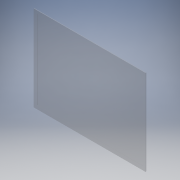
# Autodesk Inventor part: resistive_panel_12.1
Saved by Autodesk Inventor 2017 (Build 210142000, 142)
## iProperties
Created: 2017-04-25
Part Number: resistive_panel_12.1
Material: Szkło
Document SubType Name: Modeling
Designer: Speed King
Density: 2.18 g/cm^3
Appearance: Poliwęglan — przezroczysty
Mass: 270.887 g
Surface Area: 1618.77 cm^2
Volume: 124.26 cm^3
Author: Speed King
Autodesk Inventor part; units mm, degrees
ref_plane "YZ Plane" through (0, 0, 0) normal (1, 0, 0) x (0, 1, 0)
ref_plane "XZ Plane" through (0, 0, 0) normal (0, 1, 0) x (-1, 0, 0)
ref_plane "XY Plane" through (0, 0, 0) normal (0, 0, 1) x (1, 0, 0)
sketch "Szkic1" plane through (0, 0, 0) normal (0, 1, 0) x (-1, 0, 0)
  line L0 (-161, -123.5) -> (161, -123.5)
  line L1 (161, -123.5) -> (161, 123.5)
  line L2 (161, 123.5) -> (-161, 123.5)
  line L3 (-161, 123.5) -> (-161, -123.5)
  line L4 (-161, -123.5) -> (161, 123.5) construction
  line L5 (161, -123.5) -> (-161, 123.5) construction
  point P0 (0, 0)
  dimension "d0" = 322
  dimension "d1" = 247
  constraints: 12 end point, 2 midpoint, 2 parallel, 1 horizontal, 1 perpendicular
  measures "d0" distance of L2.end L1.end
  measures "d1" distance of L1.end L0.end
extrude "Wyciągnięcie proste1" add sketch "Szkic1" along normal blind 2
sketch "Szkic2" plane through (0, 2, 0) normal (0, 1, 0) x (1, 0, 0)
  line L0 (161, 123.5) -> (-161, 123.5) projected
  line L1 (-161, 123.5) -> (-161, -123.5) projected
  line L2 (-161, -123.5) -> (161, -123.5) projected
  line L3 (161, -123.5) -> (161, 123.5) projected
  line L4 (152, 114) -> (-152, 114)
  line L5 (-152, 114) -> (-152, -114)
  line L6 (-152, -114) -> (152, -114)
  line L7 (152, -114) -> (152, 114)
  line L8 (152, 114) -> (-152, -114) construction
  line L9 (-152, 114) -> (152, -114) construction
  point P0 (0, 0)
  dimension "d11" = 9
  dimension "d12" = 9
  dimension "d13" = 9.5
  dimension "d14" = 9.5
  constraints: 12 end point, 2 midpoint, 2 parallel, 1 horizontal, 1 perpendicular
  measures "d11" distance between parallel lines of L1 L5
  measures "d12" distance between parallel lines of L3 L7
  measures "d13" distance between parallel lines of L0 L4
  measures "d14" distance between parallel lines of L2 L6
extrude "Wyciągnięcie proste3" cut sketch "Szkic2" against normal blind 0.5 contours L7 L6 L5 L4
equation "\"d14\" = d13"
